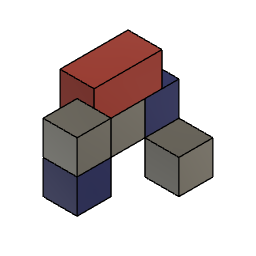
test_color (Autodesk Fusion 360 design; units mm, degrees)
Autodesk Fusion 360 part; units mm, degrees
box "Grundkörper Quader1" add length 50 width 50 height 50 placed x (0, -1, 0) y (1, 0, 0) z (0, 0, 1) at (0, 0, 0) makes body 1
copy_body "Körper->Berechn1" bodies 1 removing the originals makes body 2 in component "base_link"
box "Grundkörper Quader2" add length 50 width 50 height 50 placed x (0, 1, 0) y (-1, 0, 0) z (0, 0, 1) at (0, 50, 0) separate body makes body 3
copy_body "Körper->Berechn2" bodies 3 removing the originals makes body 4 in component "Component"
move_body "Verschieben1" bodies 4 to x (1, 0, 0) y (0, 1, 0) z (0, 0, 1) at (0, 50, 0) in component "Component"
box "Grundkörper Quader3" add length 50 width 50 height 50 placed x (0, 1, 0) y (-1, 0, 0) z (0, 0, 1) at (100, 50, 0) separate body makes body 5
copy_body "Körper->Berechn3" bodies 5 removing the originals makes body 6 in component "Component'"
box "Grundkörper Quader4" add length 50 width 50 height 50 placed x (0, 1, 0) y (-1, 0, 0) z (0, 0, 1) at (150, 50, 0) separate body makes body 7
copy_body "Körper->Berechn4" bodies 7 removing the originals makes body 8 in component "Component''"
box "Grundkörper Quader1'" add length 50 width 50 height 100 placed x (0, 1, 0) y (-1, 0, 0) z (0, 0, 1) at (150, -150, 0) separate body makes body 9 in component "Component'"
copy_body "Körper->Berechn1'" bodies 9 removing the originals makes body 10 in component "Component'''"
box "Grundkörper Quader5" add length 50 width 50 height 50 placed x (0, 0, -1) y (-1, 0, 0) z (0, 1, 0) at (0, 0, -50) separate body makes body 11
copy_body "Körper->Berechn5" bodies 11 removing the originals makes body 12 in component "Component''''"
component "base_link" placed x (1, 0, 0) y (0, 1, 0) z (0, 0, 1) at (0, 0, 0)
component "Component'" placed x (1, 0, 0) y (0, 1, 0) z (0, 0, 1) at (0, 0, 0)
component "Component'''" placed x (1, 0, 0) y (0, 0, -1) z (0, 1, 0) at (-150, 25, -50)
component "Component''''" placed x (1, 0, 0) y (0, -1, 0) z (0, 0, -1) at (50, 0, 0)
component "Component" placed x (1, 0, 0) y (0, 1, 0) z (0, 0, 1) at (0, 0, 0) in component "base_link"
component "Component''" placed x (1, 0, 0) y (0, 1, 0) z (0, 0, 1) at (-150, 0, 0) in component "Component'"
